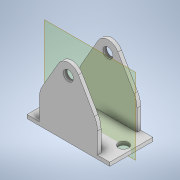
# Autodesk Inventor part: mounter
Saved by Autodesk Inventor 2022 (Build 260153000, 153)
## iProperties
Created: 2022-04-20
Part Number: mounter
Material: Generic
Document SubType Name: Modeling
Designer: Yazawa
Density: 1 g/cm^3
Appearance: Default
Author: Yazawa
Autodesk Inventor part; units mm, degrees
ref_plane "YZ Plane" through (0, 0, 0) normal (1, 0, 0) x (0, 1, 0)
ref_plane "XZ Plane" through (0, 0, 0) normal (0, 1, 0) x (-1, 0, 0)
ref_plane "XY Plane" through (0, 0, 0) normal (0, 0, 1) x (1, 0, 0)
sketch "スケッチ1" plane through (0, 0, 0) normal (0, 1, 0) x (-1, 0, 0)
  line L0 (18.5, 9.65) -> (-18.5, 9.65)
  line L1 (-18.5, 9.65) -> (-18.5, -9.65)
  line L2 (-18.5, -9.65) -> (18.5, -9.65)
  line L3 (18.5, -9.65) -> (18.5, 9.65)
  line L4 (0, 9.65) -> (0, -9.65)
  circle A0 centre (15, 0) radius 2.25
  circle A1 centre (-15, 0) radius 2.25
  point P0 (0, 0)
  point P1 (-15, 0)
  point P2 (0, 0)
  dimension "d0" = 37
  dimension "d1" = 19.3
  dimension "d2" = 30
  dimension "d3" = 4.5
  constraints: 10 end point, 3 midpoint, 2 centre point, 2 coincident, 2 parallel, 2 symmetric about line, 1 horizontal, 1 horizontal alignment, 1 perpendicular, 1 other
  measures "d0" distance of L1.end L2.end
  measures "d1" distance of L0.end L1.end
  measures "d2" distance of point (-15, 0) point (15, 0)
  measures "d3" diameter of A0
extrude "押し出し1" add sketch "スケッチ1" along normal blind 1.6
sketch "スケッチ2" plane through (-18.5, 0, 9.65) normal (0, 0, 1) x (1, 0, 0)
  line L0 (0, 0) -> (0, 1.6) projected
  line L1 (5.5, 1.6) -> (5.5, 13.6)
  line L2 (5.5, 13.6) -> (14.0688, 28.4417)
  line L3 (22.9312, 28.4417) -> (31.5, 13.6)
  line L4 (31.5, 13.6) -> (31.5, 1.6)
  line L5 (13.6056, 31) -> (23.0857, 31) construction
  line L6 (0, 0) -> (37, 0) projected
  arc A0 (22.9312, 28.4417) -> (14.0688, 28.4417) centre (18.5, 25.8833) ccw
  line L7 (37, 0) -> (37, 1.6) projected
  line L8 (0, 1.6) -> (37, 1.6) construction
  line L9 (31.5, 1.6) -> (37, 1.6) construction
  line L10 (5.5, 1.6) -> (0, 1.6) construction
  line L11 (5.5, 1.6) -> (31.5, 1.6)
  point P0 (18.5, 0)
  point P1 (18.5, 35.8969)
  point P2 (18.5, 0)
  dimension "d6" = 12
  dimension "d7" = 31
  dimension "d14" = 26
  dimension "d15" = 60
  constraints: 16 end point, 3 tangent, 2 collinear, 2 equal length, 2 point on circle, 2 vertical, 2 vertical alignment, 1 centre point, 1 horizontal, 1 midpoint, 1 point on line, 1 other
  measures "d6" distance of L3.end L4.end
  measures "d7" distance between parallel lines of L6 L5
  measures "d14" distance between parallel lines of L1 L4
  measures "d15" angle of L3 L2
extrude "押し出し2" add sketch "スケッチ2" against normal up to surface (19.3 mm away)
sketch "スケッチ3" plane through (18.5, 0, 9.65) normal (1, 0, 0) x (0, 0, -1)
  line L0 (0, 13.6) -> (0, 28.4417) projected
  line L1 (0, 0) -> (0, 1.6) projected
  line L2 (0, 0) -> (19.3, 0) projected
  line L3 (19.3, 0) -> (19.3, 1.6) projected
  line L4 (19.3, 13.6) -> (19.3, 28.4417) projected
  line L5 (19.3, 31) -> (19.3, 28.4417) projected
  line L6 (0, 31) -> (0, 28.4417) projected
  line L7 (1.6, 31) -> (1.6, 28.6547)
  line L8 (1.6, 28.6547) -> (1.6, 13.6)
  line L9 (1.6, 13.6) -> (1.6, 1.6)
  line L10 (1.6, 1.6) -> (17.7, 1.6)
  line L11 (17.7, 1.6) -> (17.7, 13.6)
  line L12 (17.7, 13.6) -> (17.7, 28.6547)
  line L13 (17.7, 28.6547) -> (17.7, 31)
  line L14 (1.6, 31) -> (17.7, 31)
  line L15 (0, 31) -> (19.3, 31) projected
  point P0 (9.65, 0)
  dimension "d10" = 1.6
  constraints: 16 end point, 1 collinear, 6 other
  measures "d10" distance between parallel lines of L0 L8
extrude "押し出し3" cut sketch "スケッチ3" against normal through all
fillet "フィレット1" radius 10 4 edges at (13, 13.6, -8.85) (13, 13.6, 8.85) (-13, 13.6, -8.85) (-13, 13.6, 8.85)
sketch "スケッチ4" plane through (18.5, 0, -9.65) normal (0, 0, -1) x (-1, 0, 0)
  arc A0 (22.9312, 28.4417) -> (14.0688, 28.4417) centre (18.5, 25.8833) ccw projected
  point P0 (18.5, 0)
  constraints: 1 coincident
hole "穴1" at (0, 25.8833, -9.65) direction (0, 0, 1) diameter 4.5 depth 19.3
ref_plane "作業平面1" through (18.5, 0, 0) normal (0, 0, -1) x (-1, 0, 0)
